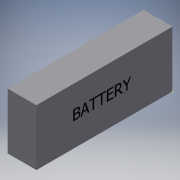
# Autodesk Inventor part: battery
Saved by Autodesk Inventor 2017 (Build 210142000, 142)
## iProperties
Created: 2017-09-05
Part Number: battery
Material: Generic
Document SubType Name: Modeling
Designer: Hp
Density: 1 g/cm^3
Appearance: Default
Author: Hp
Autodesk Inventor part; units mm, degrees
ref_plane "YZ Plane" through (0, 0, 0) normal (1, 0, 0) x (0, 1, 0)
ref_plane "XZ Plane" through (0, 0, 0) normal (0, 1, 0) x (-1, 0, 0)
ref_plane "XY Plane" through (0, 0, 0) normal (0, 0, 1) x (1, 0, 0)
sketch "Sketch1" plane through (0, 0, 0) normal (0, 0, 1) x (1, 0, 0)
  line L0 (0, 0) -> (17, 0)
  line L1 (17, 0) -> (17, 33)
  line L2 (17, 33) -> (0, 33)
  line L3 (0, 33) -> (0, 0)
  dimension "d0" = 17
  dimension "d1" = 33
  constraints: 8 end point, 2 parallel, 1 horizontal, 1 perpendicular
  measures "d0" distance of L2.end L1.end
  measures "d1" distance of L1.end L0.end
extrude "Extrusion1" add sketch "Sketch1" along normal blind 80
sketch "Sketch2" plane through (17, 0, 0) normal (1, 0, 0) x (0, 0, -1)
  line L0 (-58.9218, 20.0077) -> (-22.2104, 20.0077) construction
  line L1 (-22.2104, 20.0077) -> (-22.2104, 11.5641) construction
  line L2 (-22.2104, 11.5641) -> (-58.9218, 11.5641) construction
  line L3 (-58.9218, 11.5641) -> (-58.9218, 20.0077) construction
  point P0 (0, 0)
  constraints: 2 other
body "Solid1"
